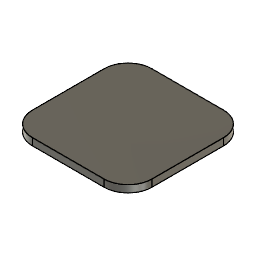
nfc tag sticker (Autodesk Fusion 360 design; units mm, degrees)
part number: 2026-06-04-14-09-21-683
Autodesk Fusion 360 part; units mm, degrees
note: some values were not read from the file. Set by a fixed rule: which sketch regions a step uses.
sketch "Sketch1" plane through (0, 0, 0) normal (0, 0, 1) x (1, 0, 0)
  circle A0 centre (0, 0) radius 12.5
  line L0 (0, 0) -> (-25, 0)
  line L1 (-25, 25) -> (25, 25)
  line L2 (25, 25) -> (25, -25)
  line L3 (25, -25) -> (-25, -25)
  line L4 (-25, -25) -> (-25, 25)
  dimension "d1" = 25
  constraint coincident A0.centre L0.start
  constraint horizontal L0
  constraint horizontal L1
  constraint vertical L2
  constraint horizontal L3
  constraint vertical L4
  measures "d1" diameter of A0
extrude "Extrude1" add sketch "Sketch1" along normal blind 3 contours A0 | L1 L2 L3 L4
extrude "Extrude2" cut sketch "Sketch1" along normal blind 0.5 contours A0
fillet "Fillet1" radius 10 4 edges at (25, -25, 1.5) (25, 25, 1.5) (-25, 25, 1.5) (-25, -25, 1.5)
sketch "Sketch2" plane through (0, 0, 0) normal (0, 0, 1) x (1, 0, 0)
